Autodesk Fusion 360 part; units mm, degrees
(part 6 of 7)
  spline S1026 degree 3 poles (3.9203, 2.2114) (3.8474, 2.0466) (3.8249, 1.9911) (3.7503, 1.7846) knots 0 0 0 0 1 1 1 1
  spline S1027 degree 3 poles (3.7503, 1.7846) (3.687, 1.6094) (3.6722, 1.5782) (3.6245, 1.5071) knots 0 0 0 0 1 1 1 1
  spline S1028 degree 3 poles (3.6245, 1.5071) (3.556, 1.4056) (3.4025, 1.1263) (3.386, 1.0742) knots 0 0 0 0 1 1 1 1
  spline S1029 degree 3 poles (3.386, 1.0742) (3.3825, 1.0629) (3.3738, 1.0395) (3.3669, 1.0222) knots 0 0 0 0 1 1 1 1
  line L131 (3.3669, 1.0222) -> (3.3539, 0.9918)
  line L132 (3.3539, 0.9918) -> (3.3261, 1.0603)
  spline S1030 degree 3 poles (3.3261, 1.0603) (3.3114, 1.0985) (3.2776, 1.1688) (3.2524, 1.2165) knots 0 0 0 0 1 1 1 1
  spline S1031 degree 3 poles (-1.6928, 1.1289) (-1.6928, 1.1306) (-1.6858, 1.1375) (-1.678, 1.1436) knots 0 0 0 0 1 1 1 1
  spline S1032 degree 3 poles (-1.678, 1.1436) (-1.6641, 1.1549) (-1.6633, 1.154) (-1.6746, 1.1401) knots 0 0 0 0 1 1 1 1
  spline S1033 degree 3 poles (-1.6746, 1.1401) (-1.6858, 1.1263) (-1.6928, 1.1219) (-1.6928, 1.1289) knots 0 0 0 0 1 1 1 1
  spline S1034 degree 3 poles (-1.6494, 1.1636) (-1.6494, 1.1653) (-1.6425, 1.1722) (-1.6347, 1.1783) knots 0 0 0 0 1 1 1 1
  spline S1035 degree 3 poles (-1.6347, 1.1783) (-1.6208, 1.1896) (-1.6199, 1.1887) (-1.6312, 1.1748) knots 0 0 0 0 1 1 1 1
  spline S1036 degree 3 poles (-1.6312, 1.1748) (-1.6425, 1.161) (-1.6494, 1.1566) (-1.6494, 1.1636) knots 0 0 0 0 1 1 1 1
  spline S1037 degree 3 poles (2.0458, 2.7969) (1.9556, 2.8646) (1.7275, 2.973) (1.6164, 2.9999) knots 0 0 0 0 1 1 1 1
  spline S1038 degree 3 poles (1.6164, 2.9999) (1.5922, 3.0051) (1.5696, 3.0129) (1.5661, 3.0164) knots 0 0 0 0 1 1 1 1
  spline S1039 degree 3 poles (1.5661, 3.0164) (1.5618, 3.0198) (1.5679, 3.0389) (1.5783, 3.0597) knots 0 0 0 0 1 1 1 1
  spline S1040 degree 3 poles (1.5783, 3.0597) (1.5965, 3.0944) (1.5974, 3.1031) (1.5913, 3.2185) knots 0 0 0 0 1 1 1 1
  spline S1041 degree 3 poles (1.5913, 3.2185) (1.5861, 3.3312) (1.5817, 3.3711) (1.5661, 3.4197) knots 0 0 0 0 1 1 1 1
  spline S1042 degree 3 poles (1.5661, 3.4197) (1.5601, 3.4362) (1.5635, 3.4371) (1.6711, 3.4336) knots 0 0 0 0 1 1 1 1
  line L133 (1.6711, 3.4336) -> (1.7813, 3.431)
  line L134 (1.7813, 3.431) -> (1.8593, 3.385)
  spline S1043 degree 3 poles (1.8593, 3.385) (1.9018, 3.3607) (1.9877, 3.3122) (2.0502, 3.2783) knots 0 0 0 0 1 1 1 1
  line L135 (2.0502, 3.2783) -> (2.1629, 3.2167)
  line L136 (2.1629, 3.2167) -> (2.1829, 3.1109)
  spline S1044 degree 3 poles (2.1829, 3.1109) (2.2098, 2.9721) (2.2193, 2.8785) (2.2193, 2.7483) knots 0 0 0 0 1 1 1 1
  line L137 (2.2193, 2.7483) -> (2.2193, 2.6408)
  line L138 (2.2193, 2.6408) -> (2.156, 2.7006)
  spline S1045 degree 3 poles (2.156, 2.7006) (2.1213, 2.7336) (2.0718, 2.777) (2.0458, 2.7969) knots 0 0 0 0 1 1 1 1
  spline S1046 degree 3 poles (-1.8663, 2.7188) (-1.8663, 2.8394) (-1.8498, 3.019) (-1.8307, 3.1048) knots 0 0 0 0 1 1 1 1
  spline S1047 degree 3 poles (-1.8307, 3.1048) (-1.8125, 3.1847) (-1.8125, 3.1907) (-1.8264, 3.2055) knots 0 0 0 0 1 1 1 1
  spline S1048 degree 3 poles (-1.8264, 3.2055) (-1.8394, 3.2211) (-1.8394, 3.2228) (-1.8255, 3.235) knots 0 0 0 0 1 1 1 1
  spline S1049 degree 3 poles (-1.8255, 3.235) (-1.8038, 3.2549) (-1.5384, 3.4015) (-1.5019, 3.4145) knots 0 0 0 0 1 1 1 1
  spline S1050 degree 3 poles (-1.5019, 3.4145) (-1.4777, 3.4232) (-1.2244, 3.4449) (-1.2192, 3.4388) knots 0 0 0 0 1 1 1 1
  spline S1051 degree 3 poles (-1.2192, 3.4388) (-1.2183, 3.4379) (-1.2226, 3.4076) (-1.2296, 3.372) knots 0 0 0 0 1 1 1 1
  spline S1052 degree 3 poles (-1.2296, 3.372) (-1.2356, 3.3365) (-1.2434, 3.2619) (-1.2469, 3.2072) knots 0 0 0 0 1 1 1 1
  spline S1053 degree 3 poles (-1.2469, 3.2072) (-1.2521, 3.1118) (-1.2513, 3.1057) (-1.2296, 3.0641) knots 0 0 0 0 1 1 1 1
  spline S1054 degree 3 poles (-1.2296, 3.0641) (-1.2174, 3.0407) (-1.2087, 3.0198) (-1.2105, 3.0181) knots 0 0 0 0 1 1 1 1
  spline S1055 degree 3 poles (-1.2105, 3.0181) (-1.2122, 3.0164) (-1.2365, 3.0094) (-1.2643, 3.0025) knots 0 0 0 0 1 1 1 1
  spline S1056 degree 3 poles (-1.2643, 3.0025) (-1.3354, 2.9834) (-1.4768, 2.9262) (-1.5635, 2.8802) knots 0 0 0 0 1 1 1 1
  spline S1057 degree 3 poles (-1.5635, 2.8802) (-1.6529, 2.8333) (-1.7309, 2.7761) (-1.8012, 2.705) knots 0 0 0 0 1 1 1 1
  spline S1058 degree 3 poles (-1.8012, 2.705) (-1.8298, 2.6763) (-1.8558, 2.6529) (-1.8602, 2.6521) knots 0 0 0 0 1 1 1 1
  spline S1059 degree 3 poles (-1.8602, 2.6521) (-1.8637, 2.6521) (-1.8663, 2.6824) (-1.8663, 2.7188) knots 0 0 0 0 1 1 1 1
  spline S1060 degree 3 poles (0.6284, 2.7431) (0.5721, 2.7501) (0.4558, 2.7587) (0.3708, 2.7622) knots 0 0 0 0 1 1 1 1
  spline S1061 degree 3 poles (0.3708, 2.7622) (0.2849, 2.7648) (0.2156, 2.7692) (0.2156, 2.7718) knots 0 0 0 0 1 1 1 1
  spline S1062 degree 3 poles (0.2156, 2.7718) (0.2156, 2.7735) (0.2294, 2.8013) (0.2459, 2.8333) knots 0 0 0 0 1 1 1 1
  spline S1063 degree 3 poles (0.2459, 2.8333) (0.2806, 2.8993) (0.3578, 2.9825) (0.4073, 3.0077) knots 0 0 0 0 1 1 1 1
  spline S1064 degree 3 poles (0.4073, 3.0077) (0.5009, 3.0554) (0.6553, 3.0008) (0.7152, 2.8984) knots 0 0 0 0 1 1 1 1
  spline S1065 degree 3 poles (0.7152, 2.8984) (0.7343, 2.8663) (0.7707, 2.7544) (0.7707, 2.7293) knots 0 0 0 0 1 1 1 1
  spline S1066 degree 3 poles (0.7707, 2.7293) (0.7707, 2.7232) (0.7629, 2.7214) (0.7508, 2.7241) knots 0 0 0 0 1 1 1 1
  spline S1067 degree 3 poles (0.7508, 2.7241) (0.7403, 2.7275) (0.6857, 2.7353) (0.6284, 2.7431) knots 0 0 0 0 1 1 1 1
  spline S1068 degree 3 poles (-0.4177, 2.7414) (-0.4177, 2.77) (-0.3847, 2.8672) (-0.3647, 2.901) knots 0 0 0 0 1 1 1 1
  spline S1069 degree 3 poles (-0.3647, 2.901) (-0.324, 2.9678) (-0.2416, 3.0164) (-0.16, 3.0233) knots 0 0 0 0 1 1 1 1
  spline S1070 degree 3 poles (-0.16, 3.0233) (-0.1141, 3.0268) (-0.0993, 3.0242) (-0.0585, 3.0042) knots 0 0 0 0 1 1 1 1
  spline S1071 degree 3 poles (-0.0585, 3.0042) (-0.0317, 2.9912) (0.0065, 2.9609) (0.0308, 2.9348) knots 0 0 0 0 1 1 1 1
  spline S1072 degree 3 poles (0.0308, 2.9348) (0.0698, 2.8923) (0.1288, 2.796) (0.1288, 2.7744) knots 0 0 0 0 1 1 1 1
  spline S1073 degree 3 poles (0.1288, 2.7744) (0.1288, 2.7683) (0.0976, 2.7648) (0.0334, 2.7648) knots 0 0 0 0 1 1 1 1
  spline S1074 degree 3 poles (0.0334, 2.7648) (-0.062, 2.7648) (-0.2997, 2.744) (-0.3569, 2.7301) knots 0 0 0 0 1 1 1 1
  spline S1075 degree 3 poles (-0.3569, 2.7301) (-0.409, 2.718) (-0.4177, 2.7197) (-0.4177, 2.7414) knots 0 0 0 0 1 1 1 1
  spline S1076 degree 3 poles (1.2521, 2.8065) (1.2278, 2.816) (1.2018, 2.8264) (1.1931, 2.829) knots 0 0 0 0 1 1 1 1
  spline S1077 degree 3 poles (1.1931, 2.829) (1.1689, 2.8368) (1.1767, 2.8507) (1.2105, 2.8594) knots 0 0 0 0 1 1 1 1
  spline S1078 degree 3 poles (1.2105, 2.8594) (1.2964, 2.8811) (1.2972, 2.8811) (1.3076, 2.8507) knots 0 0 0 0 1 1 1 1
  spline S1079 degree 3 poles (1.3076, 2.8507) (1.3207, 2.8125) (1.3198, 2.7787) (1.3059, 2.7848) knots 0 0 0 0 1 1 1 1
  spline S1080 degree 3 poles (1.3059, 2.7848) (1.3007, 2.7874) (1.2755, 2.7969) (1.2521, 2.8065) knots 0 0 0 0 1 1 1 1
  spline S1081 degree 3 poles (-0.9693, 2.8056) (-0.9667, 2.8143) (-0.9624, 2.8316) (-0.9589, 2.8446) knots 0 0 0 0 1 1 1 1
  spline S1082 degree 3 poles (-0.9589, 2.8446) (-0.9546, 2.8646) (-0.9485, 2.8689) (-0.9277, 2.8689) knots 0 0 0 0 1 1 1 1
  spline S1083 degree 3 poles (-0.9277, 2.8689) (-0.8904, 2.8689) (-0.8245, 2.8507) (-0.8271, 2.8412) knots 0 0 0 0 1 1 1 1
  spline S1084 degree 3 poles (-0.8271, 2.8412) (-0.8306, 2.8316) (-0.9338, 2.7926) (-0.9581, 2.7917) knots 0 0 0 0 1 1 1 1
  spline S1085 degree 3 poles (-0.9581, 2.7917) (-0.9693, 2.7908) (-0.9728, 2.7952) (-0.9693, 2.8056) knots 0 0 0 0 1 1 1 1
  spline S1086 degree 3 poles (0.808, 2.8576) (0.8019, 2.8732) (0.8193, 3.2072) (0.8323, 3.3156) knots 0 0 0 0 1 1 1 1
  spline S1087 degree 3 poles (0.8323, 3.3156) (0.8427, 3.4076) (0.8488, 3.4327) (0.8574, 3.4327) knots 0 0 0 0 1 1 1 1
  spline S1088 degree 3 poles (0.8574, 3.4327) (0.8618, 3.4327) (0.8774, 3.4093) (0.8921, 3.3816) knots 0 0 0 0 1 1 1 1
  spline S1089 degree 3 poles (0.8921, 3.3816) (0.9234, 3.3226) (0.9381, 3.3139) (0.9676, 3.333) knots 0 0 0 0 1 1 1 1
  spline S1090 degree 3 poles (0.9676, 3.333) (0.9988, 3.3538) (1.0006, 3.3685) (0.9772, 3.4006) knots 0 0 0 0 1 1 1 1
  spline S1091 degree 3 poles (0.9772, 3.4006) (0.9381, 3.4518) (0.8835, 3.5472) (0.8835, 3.5637) knots 0 0 0 0 1 1 1 1
  spline S1092 degree 3 poles (0.8835, 3.5637) (0.8835, 3.5776) (0.9667, 3.8205) (0.9745, 3.83) knots 0 0 0 0 1 1 1 1
  spline S1093 degree 3 poles (0.9745, 3.83) (0.978, 3.8344) (1.0864, 3.7953) (1.1307, 3.7728) knots 0 0 0 0 1 1 1 1
  spline S1094 degree 3 poles (1.1307, 3.7728) (1.194, 3.7415) (1.2903, 3.673) (1.3337, 3.6288) knots 0 0 0 0 1 1 1 1
  line L139 (1.3337, 3.6288) -> (1.371, 3.5906)
  line L140 (1.371, 3.5906) -> (1.3519, 3.5056)
  spline S1095 degree 3 poles (1.3519, 3.5056) (1.3406, 3.4579) (1.3302, 3.4154) (1.3285, 3.4093) knots 0 0 0 0 1 1 1 1
  spline S1096 degree 3 poles (1.3285, 3.4093) (1.3224, 3.3937) (1.3701, 3.3729) (1.3926, 3.3816) knots 0 0 0 0 1 1 1 1
  spline S1097 degree 3 poles (1.3926, 3.3816) (1.4057, 3.3859) (1.4135, 3.4006) (1.4204, 3.4327) knots 0 0 0 0 1 1 1 1
  spline S1098 degree 3 poles (1.4204, 3.4327) (1.4256, 3.457) (1.4299, 3.4839) (1.4299, 3.4935) knots 0 0 0 0 1 1 1 1
  spline S1099 degree 3 poles (1.4299, 3.4935) (1.4299, 3.5151) (1.443, 3.5221) (1.4551, 3.5073) knots 0 0 0 0 1 1 1 1
  spline S1100 degree 3 poles (1.4551, 3.5073) (1.4612, 3.5004) (1.4777, 3.4492) (1.4915, 3.392) knots 0 0 0 0 1 1 1 1
  spline S1101 degree 3 poles (1.4915, 3.392) (1.5236, 3.2679) (1.5306, 3.13) (1.5071, 3.0944) knots 0 0 0 0 1 1 1 1
  spline S1102 degree 3 poles (1.5071, 3.0944) (1.4646, 3.0303) (1.3753, 2.9791) (1.2435, 2.9435) knots 0 0 0 0 1 1 1 1
  spline S1103 degree 3 poles (1.2435, 2.9435) (1.1203, 2.9105) (0.8601, 2.849) (0.8201, 2.8438) knots 0 0 0 0 1 1 1 1
  spline S1104 degree 3 poles (0.8201, 2.8438) (0.8167, 2.8429) (0.8106, 2.8498) (0.808, 2.8576) knots 0 0 0 0 1 1 1 1
  spline S1105 degree 3 poles (-0.6631, 2.8871) (-0.9893, 2.9652) (-1.0509, 2.9869) (-1.1168, 3.0441) knots 0 0 0 0 1 1 1 1
  spline S1106 degree 3 poles (-1.1168, 3.0441) (-1.1342, 3.0589) (-1.1515, 3.0814) (-1.1567, 3.0936) knots 0 0 0 0 1 1 1 1
  spline S1107 degree 3 poles (-1.1567, 3.0936) (-1.1827, 3.1612) (-1.1394, 3.477) (-1.0995, 3.5099) knots 0 0 0 0 1 1 1 1
  spline S1108 degree 3 poles (-1.0995, 3.5099) (-1.0847, 3.5221) (-1.0795, 3.5117) (-1.0717, 3.4492) knots 0 0 0 0 1 1 1 1
  spline S1109 degree 3 poles (-1.0717, 3.4492) (-1.0682, 3.4258) (-1.0604, 3.3998) (-1.0535, 3.3928) knots 0 0 0 0 1 1 1 1
  spline S1110 degree 3 poles (-1.0535, 3.3928) (-1.0405, 3.3798) (-0.9936, 3.3764) (-0.9867, 3.3876) knots 0 0 0 0 1 1 1 1
  spline S1111 degree 3 poles (-0.9867, 3.3876) (-0.985, 3.3911) (-0.9902, 3.4379) (-0.9988, 3.4917) knots 0 0 0 0 1 1 1 1
  spline S1112 degree 3 poles (-0.9988, 3.4917) (-1.0084, 3.5446) (-1.0136, 3.5941) (-1.011, 3.6001) knots 0 0 0 0 1 1 1 1
  spline S1113 degree 3 poles (-1.011, 3.6001) (-0.9971, 3.6366) (-0.7959, 3.7719) (-0.7091, 3.804) knots 0 0 0 0 1 1 1 1
  spline S1114 degree 3 poles (-0.7091, 3.804) (-0.6206, 3.837) (-0.631, 3.843) (-0.5929, 3.7433) knots 0 0 0 0 1 1 1 1
  spline S1115 degree 3 poles (-0.5929, 3.7433) (-0.5738, 3.6938) (-0.5521, 3.6331) (-0.5434, 3.6071) knots 0 0 0 0 1 1 1 1
  spline S1116 degree 3 poles (-0.5434, 3.6071) (-0.5287, 3.5611) (-0.5287, 3.5602) (-0.5486, 3.5247) knots 0 0 0 0 1 1 1 1
  spline S1117 degree 3 poles (-0.5486, 3.5247) (-0.5591, 3.5056) (-0.5851, 3.464) (-0.6059, 3.4336) knots 0 0 0 0 1 1 1 1
  spline S1118 degree 3 poles (-0.6059, 3.4336) (-0.6484, 3.3711) (-0.6501, 3.3633) (-0.6267, 3.3425) knots 0 0 0 0 1 1 1 1
  spline S1119 degree 3 poles (-0.6267, 3.3425) (-0.6059, 3.3234) (-0.5738, 3.3278) (-0.5617, 3.3503) knots 0 0 0 0 1 1 1 1
  spline S1120 degree 3 poles (-0.5617, 3.3503) (-0.5374, 3.3954) (-0.5165, 3.4241) (-0.5079, 3.4241) knots 0 0 0 0 1 1 1 1
  spline S1121 degree 3 poles (-0.5079, 3.4241) (-0.4975, 3.4241) (-0.4949, 3.4093) (-0.474, 3.2419) knots 0 0 0 0 1 1 1 1
  spline S1122 degree 3 poles (-0.474, 3.2419) (-0.4584, 3.1213) (-0.4567, 2.8429) (-0.4706, 2.8429) knots 0 0 0 0 1 1 1 1
  spline S1123 degree 3 poles (-0.4706, 2.8429) (-0.4758, 2.8429) (-0.5625, 2.8628) (-0.6631, 2.8871) knots 0 0 0 0 1 1 1 1
  spline S1124 degree 3 poles (0.1548, 2.8854) (0.1401, 2.9131) (0.1444, 2.921) (0.1765, 2.921) knots 0 0 0 0 1 1 1 1
  spline S1125 degree 3 poles (0.1765, 2.921) (0.2104, 2.921) (0.2164, 2.9062) (0.193, 2.8828) knots 0 0 0 0 1 1 1 1
  spline S1126 degree 3 poles (0.193, 2.8828) (0.1757, 2.8646) (0.1661, 2.8654) (0.1548, 2.8854) knots 0 0 0 0 1 1 1 1
  spline S1127 degree 3 poles (0.4463, 3.1552) (0.4775, 3.1933) (0.5053, 3.2246) (0.507, 3.2246) knots 0 0 0 0 1 1 1 1
  spline S1128 degree 3 poles (0.507, 3.2246) (0.5087, 3.2246) (0.5105, 3.1951) (0.5105, 3.1595) knots 0 0 0 0 1 1 1 1
  line L141 (0.5105, 3.1595) -> (0.5105, 3.0953)
  line L142 (0.5105, 3.0953) -> (0.4602, 3.0918)
  spline S1129 degree 3 poles (0.4602, 3.0918) (0.4333, 3.0901) (0.4055, 3.0884) (0.3994, 3.0875) knots 0 0 0 0 1 1 1 1
  spline S1130 degree 3 poles (0.3994, 3.0875) (0.3934, 3.0866) (0.4142, 3.117) (0.4463, 3.1552) knots 0 0 0 0 1 1 1 1
  line L143 (-0.1297, 3.0996) -> (-0.1661, 3.1057)
  line L144 (-0.1661, 3.1057) -> (-0.1661, 3.1647)
  spline S1131 degree 3 poles (-0.1661, 3.1647) (-0.1661, 3.1977) (-0.1644, 3.2246) (-0.1626, 3.2246) knots 0 0 0 0 1 1 1 1
  spline S1132 degree 3 poles (-0.1626, 3.2246) (-0.1566, 3.2246) (-0.0499, 3.1118) (-0.0412, 3.097) knots 0 0 0 0 1 1 1 1
  spline S1133 degree 3 poles (-0.0412, 3.097) (-0.0351, 3.0858) (-0.0386, 3.084) (-0.0629, 3.0884) knots 0 0 0 0 1 1 1 1
  spline S1134 degree 3 poles (-0.0629, 3.0884) (-0.0794, 3.0918) (-0.1089, 3.0962) (-0.1297, 3.0996) knots 0 0 0 0 1 1 1 1
  spline S1135 degree 3 poles (0.0638, 3.2089) (0.0846, 3.2705) (0.1184, 3.3373) (0.1297, 3.3373) knots 0 0 0 0 1 1 1 1
  spline S1136 degree 3 poles (0.1297, 3.3373) (0.1349, 3.3373) (0.1375, 3.3347) (0.1358, 3.3304) knots 0 0 0 0 1 1 1 1
  spline S1137 degree 3 poles (0.1358, 3.3304) (0.108, 3.274) (0.0681, 3.1873) (0.0638, 3.1725) knots 0 0 0 0 1 1 1 1
  spline S1138 degree 3 poles (0.0638, 3.1725) (0.0603, 3.1621) (0.056, 3.156) (0.0533, 3.1586) knots 0 0 0 0 1 1 1 1
  spline S1139 degree 3 poles (0.0533, 3.1586) (0.0507, 3.1604) (0.056, 3.1838) (0.0638, 3.2089) knots 0 0 0 0 1 1 1 1
  spline S1140 degree 3 poles (-0.0568, 3.2211) (-0.0603, 3.2315) (-0.0577, 3.2332) (-0.0447, 3.2289) knots 0 0 0 0 1 1 1 1
  spline S1141 degree 3 poles (-0.0447, 3.2289) (-0.0317, 3.2246) (-0.0273, 3.2272) (-0.0273, 3.2384) knots 0 0 0 0 1 1 1 1
  spline S1142 degree 3 poles (-0.0273, 3.2384) (-0.0273, 3.2471) (-0.0256, 3.2514) (-0.023, 3.2488) knots 0 0 0 0 1 1 1 1
  spline S1143 degree 3 poles (-0.023, 3.2488) (-0.0195, 3.2462) (-0.0204, 3.2341) (-0.023, 3.222) knots 0 0 0 0 1 1 1 1
  spline S1144 degree 3 poles (-0.023, 3.222) (-0.0291, 3.1985) (-0.0481, 3.1985) (-0.0568, 3.2211) knots 0 0 0 0 1 1 1 1
  spline S1145 degree 3 poles (0.1791, 3.3425) (0.1566, 3.346) (0.1401, 3.3521) (0.1427, 3.3564) knots 0 0 0 0 1 1 1 1
  spline S1146 degree 3 poles (0.1427, 3.3564) (0.1488, 3.3659) (0.2147, 3.3564) (0.2294, 3.3451) knots 0 0 0 0 1 1 1 1
  spline S1147 degree 3 poles (0.2294, 3.3451) (0.2355, 3.3399) (0.2416, 3.3278) (0.245, 3.3174) knots 0 0 0 0 1 1 1 1
  line L145 (0.245, 3.3174) -> (0.2494, 3.2983)
  line L146 (0.2494, 3.2983) -> (0.2346, 3.3174)
  spline S1148 degree 3 poles (0.2346, 3.3174) (0.2251, 3.3312) (0.2069, 3.3391) (0.1791, 3.3425) knots 0 0 0 0 1 1 1 1
  spline S1149 degree 3 poles (0.2962, 3.3998) (0.2988, 3.4058) (0.3006, 3.4015) (0.3006, 3.3894) knots 0 0 0 0 1 1 1 1
  spline S1150 degree 3 poles (0.3006, 3.3894) (0.3006, 3.3772) (0.2988, 3.3729) (0.2962, 3.3781) knots 0 0 0 0 1 1 1 1
  spline S1151 degree 3 poles (0.2962, 3.3781) (0.2945, 3.3842) (0.2945, 3.3946) (0.2962, 3.3998) knots 0 0 0 0 1 1 1 1
  spline S1152 degree 3 poles (0.1384, 3.4605) (0.1297, 3.4813) (0.1201, 3.5082) (0.1167, 3.5212) knots 0 0 0 0 1 1 1 1
  line L147 (0.1167, 3.5212) -> (0.1115, 3.5455)
  line L148 (0.1115, 3.5455) -> (0.1722, 3.5455)
  spline S1153 degree 3 poles (0.1722, 3.5455) (0.2051, 3.5455) (0.2329, 3.542) (0.2329, 3.5377) knots 0 0 0 0 1 1 1 1
  spline S1154 degree 3 poles (0.2329, 3.5377) (0.2329, 3.5203) (0.2051, 3.4544) (0.1921, 3.4397) knots 0 0 0 0 1 1 1 1
  spline S1155 degree 3 poles (0.1921, 3.4397) (0.1705, 3.4154) (0.1548, 3.4215) (0.1384, 3.4605) knots 0 0 0 0 1 1 1 1
  spline S1156 degree 3 poles (2.6096, 3.5013) (2.4596, 3.5203) (2.0337, 3.5837) (1.9122, 3.6045) knots 0 0 0 0 1 1 1 1
  line L149 (1.9122, 3.6045) -> (1.8272, 3.6192)
  line L150 (1.8272, 3.6192) -> (1.8081, 3.6652)
  spline S1157 degree 3 poles (1.8081, 3.6652) (1.7986, 3.6895) (1.7856, 3.712) (1.7795, 3.7138) knots 0 0 0 0 1 1 1 1
  spline S1158 degree 3 poles (1.7795, 3.7138) (1.7734, 3.7164) (1.75, 3.7129) (1.7275, 3.706) knots 0 0 0 0 1 1 1 1
  spline S1159 degree 3 poles (1.7275, 3.706) (1.7041, 3.699) (1.6737, 3.693) (1.6598, 3.693) knots 0 0 0 0 1 1 1 1
  spline S1160 degree 3 poles (1.6598, 3.693) (1.6312, 3.693) (1.5939, 3.7094) (1.5887, 3.7233) knots 0 0 0 0 1 1 1 1
  spline S1161 degree 3 poles (1.5887, 3.7233) (1.5843, 3.7372) (1.7396, 3.9723) (1.8402, 4.105) knots 0 0 0 0 1 1 1 1
  spline S1162 degree 3 poles (1.8402, 4.105) (1.9556, 4.255) (2.0224, 4.3314) (2.0554, 4.3487) knots 0 0 0 0 1 1 1 1
  spline S1163 degree 3 poles (2.0554, 4.3487) (2.0692, 4.3557) (2.195, 4.3904) (2.3347, 4.4259) knots 0 0 0 0 1 1 1 1
  spline S1164 degree 3 poles (2.3347, 4.4259) (2.4735, 4.4615) (2.6226, 4.4997) (2.666, 4.5118) knots 0 0 0 0 1 1 1 1
  line L151 (2.666, 4.5118) -> (2.7441, 4.5326)
  line L152 (2.7441, 4.5326) -> (2.9653, 4.314)
  spline S1165 degree 3 poles (2.9653, 4.314) (3.0867, 4.1935) (3.2082, 4.0746) (3.2342, 4.0495) knots 0 0 0 0 1 1 1 1
  line L153 (3.2342, 4.0495) -> (3.281, 4.0035)
  line L154 (3.281, 4.0035) -> (3.0347, 3.7606)
  spline S1166 degree 3 poles (3.0347, 3.7606) (2.8985, 3.6262) (2.7753, 3.5099) (2.7614, 3.5013) knots 0 0 0 0 1 1 1 1
  spline S1167 degree 2 poles (2.7614, 3.5013) (2.7467, 3.4917) (2.7354, 3.4848) knots 0 0 0 1 1 1
  spline S1168 degree 2 poles (2.7354, 3.4848) (2.679, 3.4926) (2.6096, 3.5013) knots 0 0 0 1 1 1
  spline S1169 degree 3 poles (-2.7146, 3.7433) (-2.8586, 3.8855) (-2.9766, 4.0044) (-2.9766, 4.007) knots 0 0 0 0 1 1 1 1
  spline S1170 degree 3 poles (-2.9766, 4.007) (-2.9766, 4.0104) (-2.9713, 4.0182) (-2.9644, 4.0243) knots 0 0 0 0 1 1 1 1
  spline S1171 degree 3 poles (-2.9644, 4.0243) (-2.9575, 4.0304) (-2.8404, 4.1466) (-2.7042, 4.2819) knots 0 0 0 0 1 1 1 1
  line L155 (-2.7042, 4.2819) -> (-2.457, 4.5283)
  line L156 (-2.457, 4.5283) -> (-2.4197, 4.5222)
  spline S1172 degree 3 poles (-2.4197, 4.5222) (-2.3225, 4.5075) (-1.8524, 4.4008) (-1.7769, 4.3765) knots 0 0 0 0 1 1 1 1
  spline S1173 degree 3 poles (-1.7769, 4.3765) (-1.6772, 4.3444) (-1.6746, 4.3418) (-1.5141, 4.1336) knots 0 0 0 0 1 1 1 1
  spline S1174 degree 3 poles (-1.5141, 4.1336) (-1.3614, 3.935) (-1.2417, 3.7537) (-1.2417, 3.7207) knots 0 0 0 0 1 1 1 1
  spline S1175 degree 3 poles (-1.2417, 3.7207) (-1.2417, 3.7077) (-1.2773, 3.693) (-1.3068, 3.693) knots 0 0 0 0 1 1 1 1
  spline S1176 degree 3 poles (-1.3068, 3.693) (-1.3189, 3.693) (-1.3458, 3.699) (-1.3684, 3.7068) knots 0 0 0 0 1 1 1 1
  spline S1177 degree 3 poles (-1.3684, 3.7068) (-1.4195, 3.7242) (-1.4421, 3.7138) (-1.4681, 3.6617) knots 0 0 0 0 1 1 1 1
  spline S1178 degree 3 poles (-1.4681, 3.6617) (-1.4846, 3.627) (-1.4889, 3.6244) (-1.5262, 3.6192) knots 0 0 0 0 1 1 1 1
  spline S1179 degree 3 poles (-1.5262, 3.6192) (-1.5488, 3.6166) (-1.6043, 3.608) (-1.6494, 3.601) knots 0 0 0 0 1 1 1 1
  spline S1180 degree 3 poles (-1.6494, 3.601) (-1.6945, 3.5932) (-1.7691, 3.5819) (-1.8142, 3.5759) knots 0 0 0 0 1 1 1 1
  spline S1181 degree 3 poles (-1.8142, 3.5759) (-1.8593, 3.5698) (-1.9478, 3.5559) (-2.0094, 3.5464) knots 0 0 0 0 1 1 1 1
  spline S1182 degree 3 poles (-2.0094, 3.5464) (-2.1482, 3.5238) (-2.2228, 3.5134) (-2.352, 3.4987) knots 0 0 0 0 1 1 1 1
  spline S1183 degree 3 poles (-2.352, 3.4987) (-2.4067, 3.4917) (-2.4518, 3.4865) (-2.4518, 3.4856) knots 0 0 0 0 1 1 1 1
  spline S1184 degree 2 poles (-2.4518, 3.4856) (-2.5706, 3.601) (-2.7146, 3.7433) knots 0 0 0 1 1 1
  spline S1185 degree 3 poles (-1.4039, 3.5056) (-1.4143, 3.516) (-1.4143, 3.5785) (-1.4048, 3.5967) knots 0 0 0 0 1 1 1 1
  spline S1186 degree 3 poles (-1.4048, 3.5967) (-1.3848, 3.634) (-1.371, 3.6366) (-1.3241, 3.6088) knots 0 0 0 0 1 1 1 1
  spline S1187 degree 3 poles (-1.3241, 3.6088) (-1.2998, 3.5949) (-1.2565, 3.5785) (-1.227, 3.5724) knots 0 0 0 0 1 1 1 1
  spline S1188 degree 3 poles (-1.227, 3.5724) (-1.1671, 3.5594) (-1.1628, 3.5464) (-1.2105, 3.5221) knots 0 0 0 0 1 1 1 1
  spline S1189 degree 3 poles (-1.2105, 3.5221) (-1.2521, 3.5004) (-1.3874, 3.4882) (-1.4039, 3.5056) knots 0 0 0 0 1 1 1 1
  spline S1190 degree 3 poles (1.5869, 3.5203) (1.5401, 3.5282) (1.5132, 3.542) (1.521, 3.5542) knots 0 0 0 0 1 1 1 1
  spline S1191 degree 3 poles (1.521, 3.5542) (1.5228, 3.5576) (1.547, 3.5628) (1.5748, 3.5663) knots 0 0 0 0 1 1 1 1
  spline S1192 degree 3 poles (1.5748, 3.5663) (1.6069, 3.5698) (1.6433, 3.5828) (1.678, 3.6019) knots 0 0 0 0 1 1 1 1
  spline S1193 degree 3 poles (1.678, 3.6019) (1.7084, 3.6192) (1.7344, 3.6296) (1.7361, 3.6262) knots 0 0 0 0 1 1 1 1
  spline S1194 degree 3 poles (1.7361, 3.6262) (1.744, 3.6123) (1.7518, 3.5195) (1.7466, 3.5099) knots 0 0 0 0 1 1 1 1
  spline S1195 degree 3 poles (1.7466, 3.5099) (1.7405, 3.5004) (1.6789, 3.5039) (1.5869, 3.5203) knots 0 0 0 0 1 1 1 1
  spline S1196 degree 3 poles (0.7967, 3.6123) (0.7967, 3.621) (0.8297, 3.6756) (0.8349, 3.6756) knots 0 0 0 0 1 1 1 1
  spline S1197 degree 3 poles (0.8349, 3.6756) (0.8392, 3.6756) (0.8271, 3.6279) (0.8184, 3.6149) knots 0 0 0 0 1 1 1 1
  spline S1198 degree 3 poles (0.8184, 3.6149) (0.8123, 3.6045) (0.7967, 3.6027) (0.7967, 3.6123) knots 0 0 0 0 1 1 1 1
  spline S1199 degree 3 poles (-0.4871, 3.6591) (-0.4983, 3.6799) (-0.4983, 3.6843) (-0.4836, 3.6843) knots 0 0 0 0 1 1 1 1
  spline S1200 degree 3 poles (-0.4836, 3.6843) (-0.4766, 3.6843) (-0.4671, 3.673) (-0.4628, 3.6591) knots 0 0 0 0 1 1 1 1
  spline S1201 degree 3 poles (-0.4628, 3.6591) (-0.455, 3.6374) (-0.4558, 3.634) (-0.4662, 3.6383) knots 0 0 0 0 1 1 1 1
  spline S1202 degree 3 poles (-0.4662, 3.6383) (-0.4732, 3.6409) (-0.4827, 3.6505) (-0.4871, 3.6591) knots 0 0 0 0 1 1 1 1
  spline S1203 degree 3 poles (-1.181, 3.6557) (-1.1827, 3.6574) (-1.1801, 3.6661) (-1.1741, 3.6739) knots 0 0 0 0 1 1 1 1
  spline S1204 degree 3 poles (-1.1741, 3.6739) (-1.1107, 3.7615) (-1.1116, 3.7693) (-1.1957, 3.8734) knots 0 0 0 0 1 1 1 1
  spline S1205 degree 3 poles (-1.1957, 3.8734) (-1.2513, 3.9419) (-1.2426, 3.9506) (-1.0899, 3.9801) knots 0 0 0 0 1 1 1 1
  spline S1206 degree 3 poles (-1.0899, 3.9801) (-0.9425, 4.0078) (-0.8982, 4.0425) (-0.8783, 4.144) knots 0 0 0 0 1 1 1 1
  line L157 (-0.8783, 4.144) -> (-0.8679, 4.1978)
  line L158 (-0.8679, 4.1978) -> (-0.8193, 4.2186)
  spline S1207 degree 3 poles (-0.8193, 4.2186) (-0.7924, 4.2308) (-0.7646, 4.2394) (-0.7568, 4.2377) knots 0 0 0 0 1 1 1 1
  spline S1208 degree 3 poles (-0.7568, 4.2377) (-0.7464, 4.236) (-0.7325, 4.1935) (-0.7022, 4.0746) knots 0 0 0 0 1 1 1 1
  spline S1209 degree 3 poles (-0.7022, 4.0746) (-0.6796, 3.9861) (-0.6614, 3.9116) (-0.6614, 3.9072) knots 0 0 0 0 1 1 1 1
  spline S1210 degree 3 poles (-0.6614, 3.9072) (-0.6605, 3.9037) (-0.6709, 3.9011) (-0.6831, 3.9011) knots 0 0 0 0 1 1 1 1
  spline S1211 degree 3 poles (-0.6831, 3.9011) (-0.6961, 3.9011) (-0.7299, 3.8907) (-0.7586, 3.8777) knots 0 0 0 0 1 1 1 1
  spline S1212 degree 3 poles (-0.7586, 3.8777) (-0.8097, 3.8543) (-0.8106, 3.8543) (-0.8227, 3.8708) knots 0 0 0 0 1 1 1 1
  spline S1213 degree 3 poles (-0.8227, 3.8708) (-0.8783, 3.9515) (-0.8921, 3.9662) (-0.913, 3.9662) knots 0 0 0 0 1 1 1 1
  spline S1214 degree 3 poles (-0.913, 3.9662) (-0.9303, 3.9662) (-0.9338, 3.9619) (-0.9364, 3.935) knots 0 0 0 0 1 1 1 1
  spline S1215 degree 3 poles (-0.9364, 3.935) (-0.9381, 3.9098) (-0.9329, 3.8951) (-0.9086, 3.863) knots 0 0 0 0 1 1 1 1
  spline S1216 degree 3 poles (-0.9086, 3.863) (-0.8913, 3.8413) (-0.8774, 3.8196) (-0.8774, 3.8161) knots 0 0 0 0 1 1 1 1
  spline S1217 degree 3 poles (-0.8774, 3.8161) (-0.8774, 3.8127) (-0.9034, 3.7927) (-0.9355, 3.771) knots 0 0 0 0 1 1 1 1
  spline S1218 degree 3 poles (-0.9355, 3.771) (-0.9676, 3.7493) (-1.0153, 3.7138) (-1.0422, 3.6921) knots 0 0 0 0 1 1 1 1
  spline S1219 degree 3 poles (-1.0422, 3.6921) (-1.0691, 3.6695) (-1.0986, 3.6496) (-1.1081, 3.647) knots 0 0 0 0 1 1 1 1
  spline S1220 degree 3 poles (-1.1081, 3.647) (-1.1246, 3.6427) (-1.1732, 3.6479) (-1.181, 3.6557) knots 0 0 0 0 1 1 1 1
  spline S1221 degree 3 poles (1.4152, 3.673) (1.3814, 3.6964) (1.2513, 3.7927) (1.2356, 3.8066) knots 0 0 0 0 1 1 1 1
  spline S1222 degree 3 poles (1.2356, 3.8066) (1.2313, 3.8101) (1.24, 3.8317) (1.2547, 3.8543) knots 0 0 0 0 1 1 1 1
  spline S1223 degree 3 poles (1.2547, 3.8543) (1.2851, 3.8985) (1.2981, 3.9497) (1.2842, 3.9636) knots 0 0 0 0 1 1 1 1
  spline S1224 degree 3 poles (1.2842, 3.9636) (1.2599, 3.9879) (1.2209, 3.9549) (1.1654, 3.8621) knots 0 0 0 0 1 1 1 1
  spline S1225 degree 3 poles (1.1654, 3.8621) (1.1576, 3.8491) (1.1532, 3.85) (1.1151, 3.8699) knots 0 0 0 0 1 1 1 1
  spline S1226 degree 3 poles (1.1151, 3.8699) (1.0925, 3.8821) (1.0596, 3.8925) (1.0431, 3.8925) knots 0 0 0 0 1 1 1 1
  spline S1227 degree 3 poles (1.0431, 3.8925) (1.0275, 3.8925) (1.0136, 3.8959) (1.0136, 3.9011) knots 0 0 0 0 1 1 1 1
  spline S1228 degree 3 poles (1.0136, 3.9011) (1.0136, 3.9055) (1.0231, 3.9471) (1.0344, 3.994) knots 0 0 0 0 1 1 1 1
  spline S1229 degree 3 poles (1.0344, 3.994) (1.0465, 4.0408) (1.0622, 4.1111) (1.0708, 4.1501) knots 0 0 0 0 1 1 1 1
  spline S1230 degree 3 poles (1.0708, 4.1501) (1.0786, 4.1891) (1.0882, 4.2256) (1.0917, 4.2299) knots 0 0 0 0 1 1 1 1
  spline S1231 degree 3 poles (1.0917, 4.2299) (1.0951, 4.236) (1.1073, 4.236) (1.1307, 4.2299) knots 0 0 0 0 1 1 1 1
  spline S1232 degree 3 poles (1.1307, 4.2299) (1.2062, 4.2108) (1.207, 4.2091) (1.2348, 4.1293) knots 0 0 0 0 1 1 1 1
  spline S1233 degree 3 poles (1.2348, 4.1293) (1.2487, 4.0885) (1.266, 4.0477) (1.2729, 4.0399) knots 0 0 0 0 1 1 1 1
  spline S1234 degree 3 poles (1.2729, 4.0399) (1.2912, 4.0191) (1.3961, 3.9827) (1.4603, 3.9749) knots 0 0 0 0 1 1 1 1
  spline S1235 degree 3 poles (1.4603, 3.9749) (1.5297, 3.9662) (1.5774, 3.9471) (1.5774, 3.9272) knots 0 0 0 0 1 1 1 1
  spline S1236 degree 3 poles (1.5774, 3.9272) (1.5774, 3.9185) (1.5557, 3.8847) (1.5297, 3.8534) knots 0 0 0 0 1 1 1 1
  spline S1237 degree 3 poles (1.5297, 3.8534) (1.4959, 3.8118) (1.482, 3.7875) (1.482, 3.7693) knots 0 0 0 0 1 1 1 1
  spline S1238 degree 3 poles (1.482, 3.7693) (1.482, 3.7398) (1.4993, 3.7034) (1.5245, 3.6808) knots 0 0 0 0 1 1 1 1
  spline S1239 degree 3 poles (1.5245, 3.6808) (1.5523, 3.6557) (1.547, 3.6496) (1.4967, 3.6496) knots 0 0 0 0 1 1 1 1
  spline S1240 degree 3 poles (1.4967, 3.6496) (1.4612, 3.6496) (1.443, 3.6548) (1.4152, 3.673) knots 0 0 0 0 1 1 1 1
  spline S1241 degree 3 poles (-0.0039, 3.6973) (0.0022, 3.7155) (0.0074, 3.7138) (0.0074, 3.6921) knots 0 0 0 0 1 1 1 1
  spline S1242 degree 3 poles (0.0074, 3.6921) (0.0074, 3.6826) (0.0039, 3.6765) (-0.0013, 3.6799) knots 0 0 0 0 1 1 1 1
  spline S1243 degree 3 poles (-0.0013, 3.6799) (-0.0056, 3.6826) (-0.0074, 3.6904) (-0.0039, 3.6973) knots 0 0 0 0 1 1 1 1
  spline S1244 degree 3 poles (0.3483, 3.7207) (0.3509, 3.7277) (0.3535, 3.7251) (0.3535, 3.7155) knots 0 0 0 0 1 1 1 1
  spline S1245 degree 3 poles (0.3535, 3.7155) (0.3543, 3.706) (0.3517, 3.7008) (0.3491, 3.7042) knots 0 0 0 0 1 1 1 1
  spline S1246 degree 3 poles (0.3491, 3.7042) (0.3465, 3.7068) (0.3457, 3.7146) (0.3483, 3.7207) knots 0 0 0 0 1 1 1 1
  spline S1247 degree 3 poles (1.4698, 4.0564) (1.4048, 4.0703) (1.3458, 4.0868) (1.338, 4.0928) knots 0 0 0 0 1 1 1 1
  spline S1248 degree 3 poles (1.338, 4.0928) (1.325, 4.1041) (1.2825, 4.19) (1.2825, 4.2056) knots 0 0 0 0 1 1 1 1
  spline S1249 degree 3 poles (1.2825, 4.2056) (1.2825, 4.2099) (1.3042, 4.2455) (1.3319, 4.2845) knots 0 0 0 0 1 1 1 1
  spline S1250 degree 3 poles (1.3319, 4.2845) (1.3588, 4.3244) (1.3961, 4.38) (1.4152, 4.4086) knots 0 0 0 0 1 1 1 1
  spline S1251 degree 3 poles (1.4152, 4.4086) (1.449, 4.458) (1.6017, 4.6636) (1.6988, 4.7911) knots 0 0 0 0 1 1 1 1
  spline S1252 degree 3 poles (1.6988, 4.7911) (1.7431, 4.8484) (1.8966, 5.0262) (1.9417, 5.0722) knots 0 0 0 0 1 1 1 1
  spline S1253 degree 3 poles (1.9417, 5.0722) (2.0371, 5.1693) (2.234, 5.2751) (2.352, 5.2925) knots 0 0 0 0 1 1 1 1
  spline S1254 degree 3 poles (2.352, 5.2925) (2.457, 5.3081) (2.555, 5.2283) (2.588, 5.0999) knots 0 0 0 0 1 1 1 1
  spline S1255 degree 3 poles (2.588, 5.0999) (2.6174, 4.9872) (2.5628, 4.9082) (2.3407, 4.7408) knots 0 0 0 0 1 1 1 1
  spline S1256 degree 3 poles (2.3407, 4.7408) (2.2193, 4.6489) (2.1386, 4.576) (2.0302, 4.4563) knots 0 0 0 0 1 1 1 1
  spline S1257 degree 3 poles (2.0302, 4.4563) (1.9174, 4.334) (1.75, 4.1249) (1.6936, 4.0373) knots 0 0 0 0 1 1 1 1
  line L159 (1.6936, 4.0373) -> (1.6511, 3.9723)
  line L160 (1.6511, 3.9723) -> (1.6199, 4.0018)
  spline S1258 degree 3 poles (1.6199, 4.0018) (1.5913, 4.0295) (1.5783, 4.0339) (1.4698, 4.0564) knots 0 0 0 0 1 1 1 1
  spline S1259 degree 3 poles (-1.3579, 4.0599) (-1.5427, 4.321) (-1.8099, 4.6038) (-2.0137, 4.7564) knots 0 0 0 0 1 1 1 1
  spline S1260 degree 3 poles (-2.0137, 4.7564) (-2.143, 4.8527) (-2.1967, 4.9065) (-2.2271, 4.9724) knots 0 0 0 0 1 1 1 1
  spline S1261 degree 3 poles (-2.2271, 4.9724) (-2.2523, 5.0253) (-2.2531, 5.0661) (-2.2306, 5.1277) knots 0 0 0 0 1 1 1 1
  spline S1262 degree 3 poles (-2.2306, 5.1277) (-2.1837, 5.2526) (-2.0866, 5.315) (-1.9747, 5.2916) knots 0 0 0 0 1 1 1 1
  spline S1263 degree 3 poles (-1.9747, 5.2916) (-1.8593, 5.2673) (-1.6919, 5.1667) (-1.58, 5.0548) knots 0 0 0 0 1 1 1 1
  spline S1264 degree 3 poles (-1.58, 5.0548) (-1.4638, 4.9394) (-1.2278, 4.6437) (-1.0812, 4.4303) knots 0 0 0 0 1 1 1 1
  spline S1265 degree 3 poles (-1.0812, 4.4303) (-1.0526, 4.3895) (-1.011, 4.3296) (-0.9876, 4.2967) knots 0 0 0 0 1 1 1 1
  spline S1266 degree 3 poles (-0.9876, 4.2967) (-0.9355, 4.2238) (-0.9303, 4.1961) (-0.9572, 4.1449) knots 0 0 0 0 1 1 1 1
  spline S1267 degree 3 poles (-0.9572, 4.1449) (-0.9858, 4.0902) (-1.0084, 4.0772) (-1.1064, 4.0616) knots 0 0 0 0 1 1 1 1
  spline S1268 degree 3 poles (-1.1064, 4.0616) (-1.2027, 4.0469) (-1.2608, 4.0243) (-1.2781, 3.9974) knots 0 0 0 0 1 1 1 1
  spline S1269 degree 3 poles (-1.2781, 3.9974) (-1.2842, 3.987) (-1.292, 3.9792) (-1.2946, 3.9792) knots 0 0 0 0 1 1 1 1
  spline S1270 degree 3 poles (-1.2946, 3.9792) (-1.2981, 3.9792) (-1.3267, 4.0156) (-1.3579, 4.0599) knots 0 0 0 0 1 1 1 1
  spline S1271 degree 3 poles (0.4871, 4.4233) (0.4897, 4.4294) (0.4914, 4.4251) (0.4914, 4.4129) knots 0 0 0 0 1 1 1 1
  spline S1272 degree 3 poles (0.4914, 4.4129) (0.4914, 4.4008) (0.4897, 4.3964) (0.4871, 4.4016) knots 0 0 0 0 1 1 1 1
  spline S1273 degree 3 poles (0.4871, 4.4016) (0.4853, 4.4077) (0.4853, 4.4181) (0.4871, 4.4233) knots 0 0 0 0 1 1 1 1
  spline S1274 degree 3 poles (-0.4038, 4.7122) (-0.396, 4.7243) (-0.3882, 4.7339) (-0.3856, 4.7339) knots 0 0 0 0 1 1 1 1
  spline S1275 degree 3 poles (-0.3856, 4.7339) (-0.3812, 4.7339) (-0.3899, 4.7183) (-0.4029, 4.7009) knots 0 0 0 0 1 1 1 1
  spline S1276 degree 3 poles (-0.4029, 4.7009) (-0.4177, 4.6818) (-0.4185, 4.6896) (-0.4038, 4.7122) knots 0 0 0 0 1 1 1 1
  spline S1277 degree 3 poles (2.5593, 5.3098) (2.5125, 5.3341) (2.4917, 5.368) (2.4726, 5.4495) knots 0 0 0 0 1 1 1 1
  spline S1278 degree 3 poles (2.4726, 5.4495) (2.4622, 5.492) (2.4231, 5.6369) (2.385, 5.7704) knots 0 0 0 0 1 1 1 1
  spline S1279 degree 3 poles (2.385, 5.7704) (2.3468, 5.904) (2.3078, 6.0463) (2.2974, 6.087) knots 0 0 0 0 1 1 1 1
  spline S1280 degree 3 poles (2.2974, 6.087) (2.2878, 6.1278) (2.2774, 6.1677) (2.2748, 6.1755) knots 0 0 0 0 1 1 1 1
  spline S1281 degree 3 poles (2.2748, 6.1755) (2.2687, 6.1963) (2.3451, 6.2041) (2.4596, 6.1929) knots 0 0 0 0 1 1 1 1
  spline S1282 degree 3 poles (2.4596, 6.1929) (2.6105, 6.1781) (2.6955, 6.1538) (2.823, 6.0914) knots 0 0 0 0 1 1 1 1
  spline S1283 degree 3 poles (2.823, 6.0914) (2.9523, 6.0281) (3.0147, 5.9847) (3.1171, 5.8875) knots 0 0 0 0 1 1 1 1
  spline S1284 degree 3 poles (3.1171, 5.8875) (3.2324, 5.78) (3.3209, 5.7123) (3.5352, 5.5683) knots 0 0 0 0 1 1 1 1
  spline S1285 degree 3 poles (3.5352, 5.5683) (3.6462, 5.4946) (3.7373, 5.4304) (3.7373, 5.4261) knots 0 0 0 0 1 1 1 1
  spline S1286 degree 3 poles (3.7373, 5.4261) (3.7373, 5.4113) (3.6904, 5.4018) (3.5699, 5.3931) knots 0 0 0 0 1 1 1 1
  spline S1287 degree 3 poles (3.5699, 5.3931) (3.5022, 5.3879) (3.4155, 5.3801) (3.3773, 5.3749) knots 0 0 0 0 1 1 1 1
  spline S1288 degree 3 poles (3.3773, 5.3749) (3.3114, 5.3671) (3.2567, 5.361) (2.9262, 5.3281) knots 0 0 0 0 1 1 1 1
  spline S1289 degree 3 poles (2.9262, 5.3281) (2.8499, 5.3202) (2.758, 5.3116) (2.7224, 5.3072) knots 0 0 0 0 1 1 1 1
  spline S1290 degree 3 poles (2.7224, 5.3072) (2.6218, 5.296) (2.5845, 5.2968) (2.5593, 5.3098) knots 0 0 0 0 1 1 1 1
  spline S1291 degree 3 poles (-2.4604, 5.3194) (-2.6296, 5.3341) (-2.8117, 5.3515) (-2.9896, 5.3714) knots 0 0 0 0 1 1 1 1
  spline S1292 degree 3 poles (-2.9896, 5.3714) (-3.052, 5.3792) (-3.1552, 5.3879) (-3.2194, 5.3922) knots 0 0 0 0 1 1 1 1
  spline S1293 degree 3 poles (-3.2194, 5.3922) (-3.3357, 5.4) (-3.3842, 5.4105) (-3.3842, 5.4278) knots 0 0 0 0 1 1 1 1
  spline S1294 degree 3 poles (-3.3842, 5.4278) (-3.3842, 5.4321) (-3.301, 5.492) (-3.2003, 5.5588) knots 0 0 0 0 1 1 1 1
  spline S1295 degree 3 poles (-3.2003, 5.5588) (-2.9913, 5.6976) (-2.9124, 5.7574) (-2.7753, 5.8797) knots 0 0 0 0 1 1 1 1
  spline S1296 degree 3 poles (-2.7753, 5.8797) (-2.5637, 6.0697) (-2.3668, 6.1642) (-2.123, 6.1911) knots 0 0 0 0 1 1 1 1
  spline S1297 degree 3 poles (-2.123, 6.1911) (-2.0441, 6.2007) (-1.927, 6.2007) (-1.927, 6.1911) knots 0 0 0 0 1 1 1 1
  spline S1298 degree 3 poles (-1.927, 6.1911) (-1.927, 6.1816) (-1.9729, 6.0064) (-2.0233, 5.8268) knots 0 0 0 0 1 1 1 1
  spline S1299 degree 3 poles (-2.0233, 5.8268) (-2.051, 5.7245) (-2.09, 5.5839) (-2.1091, 5.5145) knots 0 0 0 0 1 1 1 1
  spline S1300 degree 3 poles (-2.1091, 5.5145) (-2.1525, 5.3567) (-2.1525, 5.3558) (-2.1976, 5.3237) knots 0 0 0 0 1 1 1 1
  spline S1301 degree 3 poles (-2.1976, 5.3237) (-2.2297, 5.3003) (-2.2401, 5.2968) (-2.2696, 5.3012) knots 0 0 0 0 1 1 1 1
  spline S1302 degree 3 poles (-2.2696, 5.3012) (-2.2887, 5.3038) (-2.3746, 5.3124) (-2.4604, 5.3194) knots 0 0 0 0 1 1 1 1
  spline S1303 degree 3 poles (3.7347, 5.5414) (3.6037, 5.6082) (3.327, 5.8095) (3.1882, 5.9387) knots 0 0 0 0 1 1 1 1
  spline S1304 degree 3 poles (3.1882, 5.9387) (2.993, 6.1183) (2.8091, 6.2172) (2.5958, 6.2562) knots 0 0 0 0 1 1 1 1
  spline S1305 degree 3 poles (2.5958, 6.2562) (2.5533, 6.264) (2.4492, 6.2727) (2.365, 6.2753) knots 0 0 0 0 1 1 1 1
  line L161 (2.365, 6.2753) -> (2.2106, 6.2805)
  line L162 (2.2106, 6.2805) -> (2.1178, 6.2406)
  spline S1306 degree 3 poles (2.1178, 6.2406) (2.0024, 6.192) (1.9348, 6.1816) (1.7309, 6.1816) knots 0 0 0 0 1 1 1 1
  spline S1307 degree 3 poles (1.7309, 6.1816) (1.5436, 6.1816) (1.4447, 6.1946) (1.3172, 6.2362) knots 0 0 0 0 1 1 1 1
  spline S1308 degree 3 poles (1.3172, 6.2362) (1.2122, 6.2692) (1.1472, 6.3108) (1.0491, 6.4037) knots 0 0 0 0 1 1 1 1
  spline S1309 degree 3 poles (1.0491, 6.4037) (0.8245, 6.6179) (0.6952, 6.7055) (0.5096, 6.7706) knots 0 0 0 0 1 1 1 1
  spline S1310 degree 3 poles (0.5096, 6.7706) (0.3405, 6.8296) (0.0794, 6.8374) (-0.1141, 6.7888) knots 0 0 0 0 1 1 1 1
  spline S1311 degree 3 poles (-0.1141, 6.7888) (-0.1887, 6.7697) (-0.3491, 6.6942) (-0.4281, 6.6413) knots 0 0 0 0 1 1 1 1
  spline S1312 degree 3 poles (-0.4281, 6.6413) (-0.4862, 6.6014) (-0.5729, 6.5268) (-0.7126, 6.3967) knots 0 0 0 0 1 1 1 1
  spline S1313 degree 3 poles (-0.7126, 6.3967) (-0.7846, 6.3291) (-0.8201, 6.303) (-0.8817, 6.2727) knots 0 0 0 0 1 1 1 1
  spline S1314 degree 3 poles (-0.8817, 6.2727) (-1.0596, 6.1851) (-1.3259, 6.1556) (-1.6104, 6.192) knots 0 0 0 0 1 1 1 1
  spline S1315 degree 3 poles (-1.6104, 6.192) (-1.6728, 6.1998) (-1.8055, 6.2466) (-1.8376, 6.2709) knots 0 0 0 0 1 1 1 1
  spline S1316 degree 3 poles (-1.8376, 6.2709) (-1.8489, 6.2805) (-2.1039, 6.2813) (-2.1785, 6.2727) knots 0 0 0 0 1 1 1 1
  spline S1317 degree 3 poles (-2.1785, 6.2727) (-2.2583, 6.264) (-2.3919, 6.2276) (-2.4726, 6.192) knots 0 0 0 0 1 1 1 1
  spline S1318 degree 3 poles (-2.4726, 6.192) (-2.6053, 6.1356) (-2.7111, 6.0619) (-2.856, 5.9266) knots 0 0 0 0 1 1 1 1
  spline S1319 degree 3 poles (-2.856, 5.9266) (-2.9037, 5.8815) (-2.9731, 5.8225) (-3.0095, 5.7947) knots 0 0 0 0 1 1 1 1
  spline S1320 degree 3 poles (-3.0095, 5.7947) (-3.1058, 5.7219) (-3.3565, 5.5562) (-3.3999, 5.5371) knots 0 0 0 0 1 1 1 1
  line L163 (-3.3999, 5.5371) -> (-3.4372, 5.5206)
  line L164 (-3.4372, 5.5206) -> (-3.5083, 5.544)
  spline S1321 degree 3 poles (-3.5083, 5.544) (-3.6202, 5.5822) (-3.6705, 5.6039) (-3.6705, 5.6134) knots 0 0 0 0 1 1 1 1
  spline S1322 degree 3 poles (-3.6705, 5.6134) (-3.6705, 5.6186) (-3.654, 5.6334) (-3.6341, 5.6464) knots 0 0 0 0 1 1 1 1
  spline S1323 degree 3 poles (-3.6341, 5.6464) (-3.6132, 5.6594) (-3.5811, 5.6802) (-3.5621, 5.6941) knots 0 0 0 0 1 1 1 1
  spline S1324 degree 3 poles (-3.5621, 5.6941) (-3.543, 5.7071) (-3.4883, 5.7453) (-3.4406, 5.7782) knots 0 0 0 0 1 1 1 1
  spline S1325 degree 3 poles (-3.4406, 5.7782) (-3.3929, 5.8112) (-3.3079, 5.8719) (-3.2515, 5.9127) knots 0 0 0 0 1 1 1 1
  spline S1326 degree 3 poles (-3.2515, 5.9127) (-2.9748, 6.1139) (-2.9219, 6.1504) (-2.8248, 6.2033) knots 0 0 0 0 1 1 1 1
  spline S1327 degree 3 poles (-2.8248, 6.2033) (-2.6678, 6.2883) (-2.4604, 6.3516) (-2.2783, 6.369) knots 0 0 0 0 1 1 1 1
  spline S1328 degree 3 poles (-2.2783, 6.369) (-2.2037, 6.3759) (-2.0094, 6.3611) (-1.9443, 6.3429) knots 0 0 0 0 1 1 1 1
  spline S1329 degree 3 poles (-1.9443, 6.3429) (-1.9183, 6.3351) (-1.8819, 6.3273) (-1.8645, 6.3247) knots 0 0 0 0 1 1 1 1
  spline S1330 degree 3 poles (-1.8645, 6.3247) (-1.8463, 6.323) (-1.7899, 6.3022) (-1.7387, 6.2787) knots 0 0 0 0 1 1 1 1
  spline S1331 degree 3 poles (-1.7387, 6.2787) (-1.6867, 6.2553) (-1.6312, 6.2328) (-1.6147, 6.2276) knots 0 0 0 0 1 1 1 1
  spline S1332 degree 3 poles (-1.6147, 6.2276) (-1.554, 6.2085) (-1.4386, 6.1972) (-1.3597, 6.2033) knots 0 0 0 0 1 1 1 1
  spline S1333 degree 3 poles (-1.3597, 6.2033) (-1.109, 6.2206) (-0.8713, 6.3629) (-0.6137, 6.65) knots 0 0 0 0 1 1 1 1
  spline S1334 degree 3 poles (-0.6137, 6.65) (-0.4758, 6.8044) (-0.4142, 6.846) (-0.2641, 6.8894) knots 0 0 0 0 1 1 1 1
  spline S1335 degree 3 poles (-0.2641, 6.8894) (-0.0212, 6.9597) (0.1861, 6.9779) (0.3804, 6.9458) knots 0 0 0 0 1 1 1 1
  spline S1336 degree 3 poles (0.3804, 6.9458) (0.5365, 6.9206) (0.6276, 6.8929) (0.7325, 6.8417) knots 0 0 0 0 1 1 1 1
  spline S1337 degree 3 poles (0.7325, 6.8417) (0.8288, 6.7949) (0.8401, 6.7845) (1.0162, 6.5962) knots 0 0 0 0 1 1 1 1
  spline S1338 degree 3 poles (1.0162, 6.5962) (1.1368, 6.4678) (1.2825, 6.3507) (1.3909, 6.2935) knots 0 0 0 0 1 1 1 1
  spline S1339 degree 3 poles (1.3909, 6.2935) (1.5245, 6.2241) (1.7006, 6.192) (1.8515, 6.2094) knots 0 0 0 0 1 1 1 1
  spline S1340 degree 3 poles (1.8515, 6.2094) (1.9547, 6.2206) (1.9834, 6.2284) (2.0831, 6.2753) knots 0 0 0 0 1 1 1 1
  spline S1341 degree 3 poles (2.0831, 6.2753) (2.2202, 6.3386) (2.4526, 6.3794) (2.6131, 6.3681) knots 0 0 0 0 1 1 1 1
  spline S1342 degree 3 poles (2.6131, 6.3681) (2.9271, 6.3473) (3.1778, 6.2319) (3.6115, 5.9092) knots 0 0 0 0 1 1 1 1
  spline S1343 degree 3 poles (3.6115, 5.9092) (3.7017, 5.8424) (3.9628, 5.6594) (3.9992, 5.6369) knots 0 0 0 0 1 1 1 1
  spline S1344 degree 3 poles (3.9992, 5.6369) (4.0175, 5.6264) (4.0322, 5.6143) (4.0322, 5.6108) knots 0 0 0 0 1 1 1 1
  spline S1345 degree 3 poles (4.0322, 5.6108) (4.0322, 5.603) (3.818, 5.5293) (3.7781, 5.5241) knots 0 0 0 0 1 1 1 1
  spline S1346 degree 3 poles (3.7781, 5.5241) (3.7746, 5.5232) (3.7546, 5.5319) (3.7347, 5.5414) knots 0 0 0 0 1 1 1 1
  spline S1347 degree 3 poles (-0.8774, 5.7843) (-0.913, 5.8008) (-1.0188, 5.8537) (-1.1116, 5.9023) knots 0 0 0 0 1 1 1 1
  spline S1348 degree 3 poles (-1.1116, 5.9023) (-1.2044, 5.9509) (-1.3267, 6.0116) (-1.3831, 6.0385) knots 0 0 0 0 1 1 1 1
  spline S1349 degree 3 poles (-1.3831, 6.0385) (-1.4386, 6.0645) (-1.4846, 6.0879) (-1.4846, 6.0888) knots 0 0 0 0 1 1 1 1
  spline S1350 degree 3 poles (-1.4846, 6.0888) (-1.4846, 6.0905) (-1.4195, 6.0922) (-1.3389, 6.0922) knots 0 0 0 0 1 1 1 1
  spline S1351 degree 3 poles (-1.3389, 6.0922) (-1.2278, 6.0931) (-1.1741, 6.0975) (-1.1073, 6.1113) knots 0 0 0 0 1 1 1 1
  spline S1352 degree 3 poles (-1.1073, 6.1113) (-0.9624, 6.1426) (-0.8392, 6.1885) (-0.7638, 6.2406) knots 0 0 0 0 1 1 1 1
  spline S1353 degree 3 poles (-0.7638, 6.2406) (-0.7516, 6.2493) (-0.7022, 6.2918) (-0.6553, 6.336) knots 0 0 0 0 1 1 1 1
  spline S1354 degree 3 poles (-0.6553, 6.336) (-0.3353, 6.6327) (-0.1548, 6.7237) (0.1375, 6.735) knots 0 0 0 0 1 1 1 1
  spline S1355 degree 3 poles (0.1375, 6.735) (0.4498, 6.748) (0.6666, 6.6535) (0.9581, 6.3794) knots 0 0 0 0 1 1 1 1
  spline S1356 degree 3 poles (0.9581, 6.3794) (1.1272, 6.2206) (1.1741, 6.1911) (1.3389, 6.1408) knots 0 0 0 0 1 1 1 1
  spline S1357 degree 3 poles (1.3389, 6.1408) (1.4681, 6.1018) (1.5401, 6.0914) (1.7014, 6.0914) knots 0 0 0 0 1 1 1 1
  spline S1358 degree 3 poles (1.7014, 6.0914) (1.7813, 6.0914) (1.8411, 6.0896) (1.8359, 6.0879) knots 0 0 0 0 1 1 1 1
  spline S1359 degree 3 poles (1.8359, 6.0879) (1.822, 6.0836) (1.5288, 5.937) (1.2964, 5.819) knots 0 0 0 0 1 1 1 1
  spline S1360 degree 3 poles (1.2964, 5.819) (1.2009, 5.7704) (1.1185, 5.7323) (1.1125, 5.7331) knots 0 0 0 0 1 1 1 1
  spline S1361 degree 3 poles (1.1125, 5.7331) (1.1038, 5.7357) (0.5617, 6.2484) (0.2928, 6.5095) knots 0 0 0 0 1 1 1 1
  spline S1362 degree 3 poles (0.2928, 6.5095) (0.232, 6.5685) (0.1783, 6.6162) (0.1722, 6.6162) knots 0 0 0 0 1 1 1 1
  spline S1363 degree 3 poles (0.1722, 6.6162) (0.1661, 6.6162) (0.1236, 6.5797) (0.0776, 6.5355) knots 0 0 0 0 1 1 1 1
  spline S1364 degree 3 poles (0.0776, 6.5355) (0.0317, 6.4921) (-0.0464, 6.4167) (-0.0967, 6.369) knots 0 0 0 0 1 1 1 1
  spline S1365 degree 3 poles (-0.0967, 6.369) (-0.147, 6.3204) (-0.2442, 6.2267) (-0.3136, 6.1608) knots 0 0 0 0 1 1 1 1
  spline S1366 degree 3 poles (-0.3136, 6.1608) (-0.4897, 5.9908) (-0.5998, 5.8849) (-0.612, 5.8745) knots 0 0 0 0 1 1 1 1
  spline S1367 degree 3 poles (-0.612, 5.8745) (-0.6172, 5.8693) (-0.6562, 5.8329) (-0.6978, 5.793) knots 0 0 0 0 1 1 1 1
  line L165 (-0.6978, 5.793) -> (-0.7742, 5.721)
  line L166 (-0.7742, 5.721) -> (-0.7933, 5.7375)
  spline S1368 degree 3 poles (-0.7933, 5.7375) (-0.8037, 5.747) (-0.8418, 5.7687) (-0.8774, 5.7843) knots 0 0 0 0 1 1 1 1
  spline S1369 degree 3 poles (1.6485, 6.3065) (1.5549, 6.3343) (1.4655, 6.3889) (1.3796, 6.4722) knots 0 0 0 0 1 1 1 1
  spline S1370 degree 3 poles (1.3796, 6.4722) (1.2998, 6.5494) (1.2781, 6.5875) (1.2426, 6.7072) knots 0 0 0 0 1 1 1 1
  spline S1371 degree 3 poles (1.2426, 6.7072) (1.2244, 6.7714) (1.22, 6.8053) (1.2192, 6.8937) knots 0 0 0 0 1 1 1 1
  spline S1372 degree 3 poles (1.2192, 6.8937) (1.2174, 6.9952) (1.2192, 7.0056) (1.2408, 7.0534) knots 0 0 0 0 1 1 1 1
  spline S1373 degree 3 poles (1.2408, 7.0534) (1.338, 7.2589) (1.495, 7.4237) (1.6598, 7.4914) knots 0 0 0 0 1 1 1 1
  spline S1374 degree 3 poles (1.6598, 7.4914) (1.6988, 7.507) (1.7327, 7.514) (1.7943, 7.5166) knots 0 0 0 0 1 1 1 1
  spline S1375 degree 3 poles (1.7943, 7.5166) (1.8689, 7.52) (1.8845, 7.5174) (1.9599, 7.4923) knots 0 0 0 0 1 1 1 1
  spline S1376 degree 3 poles (1.9599, 7.4923) (2.2063, 7.4107) (2.3711, 7.2503) (2.4015, 7.0638) knots 0 0 0 0 1 1 1 1
  spline S1377 degree 3 poles (2.4015, 7.0638) (2.4162, 6.9727) (2.4006, 6.892) (2.3355, 6.7159) knots 0 0 0 0 1 1 1 1
  spline S1378 degree 3 poles (2.3355, 6.7159) (2.2618, 6.5182) (2.2323, 6.4756) (2.1109, 6.3915) knots 0 0 0 0 1 1 1 1
  spline S1379 degree 3 poles (2.1109, 6.3915) (2.0007, 6.3152) (1.9192, 6.2883) (1.7977, 6.2874) knots 0 0 0 0 1 1 1 1
  spline S1380 degree 3 poles (1.7977, 6.2874) (1.7387, 6.2866) (1.6997, 6.2918) (1.6485, 6.3065) knots 0 0 0 0 1 1 1 1
  spline S1381 degree 3 poles (-1.567, 6.2996) (-1.6728, 6.3273) (-1.8142, 6.4097) (-1.8611, 6.4713) knots 0 0 0 0 1 1 1 1
  spline S1382 degree 3 poles (-1.8611, 6.4713) (-1.8879, 6.5069) (-1.9617, 6.6535) (-1.9964, 6.7428) knots 0 0 0 0 1 1 1 1
  spline S1383 degree 3 poles (-1.9964, 6.7428) (-2.0285, 6.8226) (-2.0571, 6.9493) (-2.0571, 7.0108) knots 0 0 0 0 1 1 1 1
  spline S1384 degree 3 poles (-2.0571, 7.0108) (-2.0571, 7.0664) (-2.0259, 7.1644) (-1.9868, 7.2286) knots 0 0 0 0 1 1 1 1
  spline S1385 degree 3 poles (-1.9868, 7.2286) (-1.9322, 7.3196) (-1.8185, 7.409) (-1.6902, 7.4636) knots 0 0 0 0 1 1 1 1
  spline S1386 degree 3 poles (-1.6902, 7.4636) (-1.5202, 7.5356) (-1.3952, 7.5374) (-1.2539, 7.4706) knots 0 0 0 0 1 1 1 1
  spline S1387 degree 3 poles (-1.2539, 7.4706) (-1.1385, 7.4159) (-0.9589, 7.2156) (-0.8887, 7.062) knots 0 0 0 0 1 1 1 1
  spline S1388 degree 3 poles (-0.8887, 7.062) (-0.8679, 7.0152) (-0.867, 7.0082) (-0.8713, 6.8946) knots 0 0 0 0 1 1 1 1
  spline S1389 degree 3 poles (-0.8713, 6.8946) (-0.8757, 6.7662) (-0.8999, 6.6604) (-0.9442, 6.5797) knots 0 0 0 0 1 1 1 1
  spline S1390 degree 3 poles (-0.9442, 6.5797) (-0.9867, 6.5008) (-1.1047, 6.395) (-1.2061, 6.3429) knots 0 0 0 0 1 1 1 1
  spline S1391 degree 3 poles (-1.2061, 6.3429) (-1.3102, 6.2909) (-1.4612, 6.2727) (-1.567, 6.2996) knots 0 0 0 0 1 1 1 1
  spline S1392 degree 3 poles (1.1775, 6.5476) (1.1489, 6.5719) (1.1185, 6.6023) (1.109, 6.6162) knots 0 0 0 0 1 1 1 1
  line L167 (1.109, 6.6162) -> (1.0925, 6.6396)
  line L168 (1.0925, 6.6396) -> (1.1151, 6.6977)
  spline S1393 degree 3 poles (1.1151, 6.6977) (1.1281, 6.7289) (1.1402, 6.755) (1.1437, 6.755) knots 0 0 0 0 1 1 1 1
  spline S1394 degree 3 poles (1.1437, 6.755) (1.1472, 6.755) (1.1567, 6.7289) (1.1654, 6.696) knots 0 0 0 0 1 1 1 1
  spline S1395 degree 3 poles (1.1654, 6.696) (1.1741, 6.6639) (1.1905, 6.6162) (1.2018, 6.5901) knots 0 0 0 0 1 1 1 1
  spline S1396 degree 3 poles (1.2018, 6.5901) (1.233, 6.5199) (1.2391, 6.5034) (1.2339, 6.5034) knots 0 0 0 0 1 1 1 1
  spline S1397 degree 3 poles (1.2339, 6.5034) (1.2304, 6.5034) (1.2053, 6.5234) (1.1775, 6.5476) knots 0 0 0 0 1 1 1 1
  spline S1398 degree 3 poles (-0.8861, 6.5164) (-0.8861, 6.519) (-0.8765, 6.5398) (-0.8653, 6.5624) knots 0 0 0 0 1 1 1 1
  spline S1399 degree 3 poles (-0.8653, 6.5624) (-0.854, 6.5849) (-0.8349, 6.637) (-0.8219, 6.6786) knots 0 0 0 0 1 1 1 1
  spline S1400 degree 3 poles (-0.8219, 6.6786) (-0.8089, 6.7211) (-0.7959, 6.755) (-0.7924, 6.755) knots 0 0 0 0 1 1 1 1
  spline S1401 degree 3 poles (-0.7924, 6.755) (-0.7854, 6.755) (-0.7421, 6.6266) (-0.7481, 6.6222) knots 0 0 0 0 1 1 1 1
  spline S1402 degree 3 poles (-0.7481, 6.6222) (-0.8722, 6.5121) (-0.8861, 6.5017) (-0.8861, 6.5164) knots 0 0 0 0 1 1 1 1
  spline S1403 degree 3 poles (1.6147, -0.2902) (1.6234, -0.2885) (1.6303, -0.2781) (1.6303, -0.2659) knots 0 0 0 0 1 1 1 1
  spline S1404 degree 3 poles (1.6303, -0.2659) (1.6312, -0.2547) (1.6321, -0.2399) (1.6329, -0.2347) knots 0 0 0 0 1 1 1 1
  spline S1405 degree 3 poles (1.6329, -0.2347) (1.6338, -0.2269) (1.6052, -0.22) (1.5427, -0.213) knots 0 0 0 0 1 1 1 1
  spline S1406 degree 3 poles (1.5427, -0.213) (1.4325, -0.2009) (0.8401, -0.1723) (0.834, -0.1792) knots 0 0 0 0 1 1 1 1
  spline S1407 degree 3 poles (0.834, -0.1792) (0.8314, -0.1818) (0.8323, -0.2009) (0.8366, -0.2208) knots 0 0 0 0 1 1 1 1
  line L169 (0.8366, -0.2208) -> (0.8444, -0.2581)
  line L170 (0.8444, -0.2581) -> (1.0179, -0.2642)
  spline S1408 degree 3 poles (1.0179, -0.2642) (1.1133, -0.2677) (1.2834, -0.2755) (1.3961, -0.2816) knots 0 0 0 0 1 1 1 1
  spline S1409 degree 3 poles (1.3961, -0.2816) (1.508, -0.2876) (1.6069, -0.292) (1.6147, -0.2902) knots 0 0 0 0 1 1 1 1
  spline S1410 degree 3 poles (0.7603, 1.8948) (0.7837, 1.9035) (0.7889, 1.9399) (0.7707, 1.9746) knots 0 0 0 0 1 1 1 1
  spline S1411 degree 3 poles (0.7707, 1.9746) (0.7039, 2.1064) (0.4723, 2.188) (0.1678, 2.1871) knots 0 0 0 0 1 1 1 1
  spline S1412 degree 3 poles (0.1678, 2.1871) (-0.0299, 2.1863) (-0.1696, 2.1576) (-0.291, 2.0943) knots 0 0 0 0 1 1 1 1
  spline S1413 degree 3 poles (-0.291, 2.0943) (-0.3613, 2.057) (-0.422, 1.9989) (-0.4315, 1.9607) knots 0 0 0 0 1 1 1 1
  spline S1414 degree 3 poles (-0.4315, 1.9607) (-0.435, 1.9486) (-0.4333, 1.9304) (-0.4272, 1.9182) knots 0 0 0 0 1 1 1 1
  spline S1415 degree 3 poles (-0.4272, 1.9182) (-0.4142, 1.8887) (-0.3856, 1.8913) (-0.3674, 1.9243) knots 0 0 0 0 1 1 1 1
  spline S1416 degree 3 poles (-0.3674, 1.9243) (-0.3266, 1.9998) (-0.2529, 2.0466) (-0.1219, 2.0796) knots 0 0 0 0 1 1 1 1
  spline S1417 degree 3 poles (-0.1219, 2.0796) (-0.0455, 2.0995) (0.1245, 2.1143) (0.2112, 2.109) knots 0 0 0 0 1 1 1 1
  spline S1418 degree 3 poles (0.2112, 2.109) (0.3804, 2.0995) (0.4133, 2.096) (0.4654, 2.083) knots 0 0 0 0 1 1 1 1
  spline S1419 degree 3 poles (0.4654, 2.083) (0.4975, 2.0752) (0.5521, 2.0561) (0.5859, 2.0397) knots 0 0 0 0 1 1 1 1
  spline S1420 degree 3 poles (0.5859, 2.0397) (0.6363, 2.0154) (0.6579, 1.9989) (0.6935, 1.9555) knots 0 0 0 0 1 1 1 1
  spline S1421 degree 3 poles (0.6935, 1.9555) (0.7499, 1.8879) (0.7473, 1.8905) (0.7603, 1.8948) knots 0 0 0 0 1 1 1 1